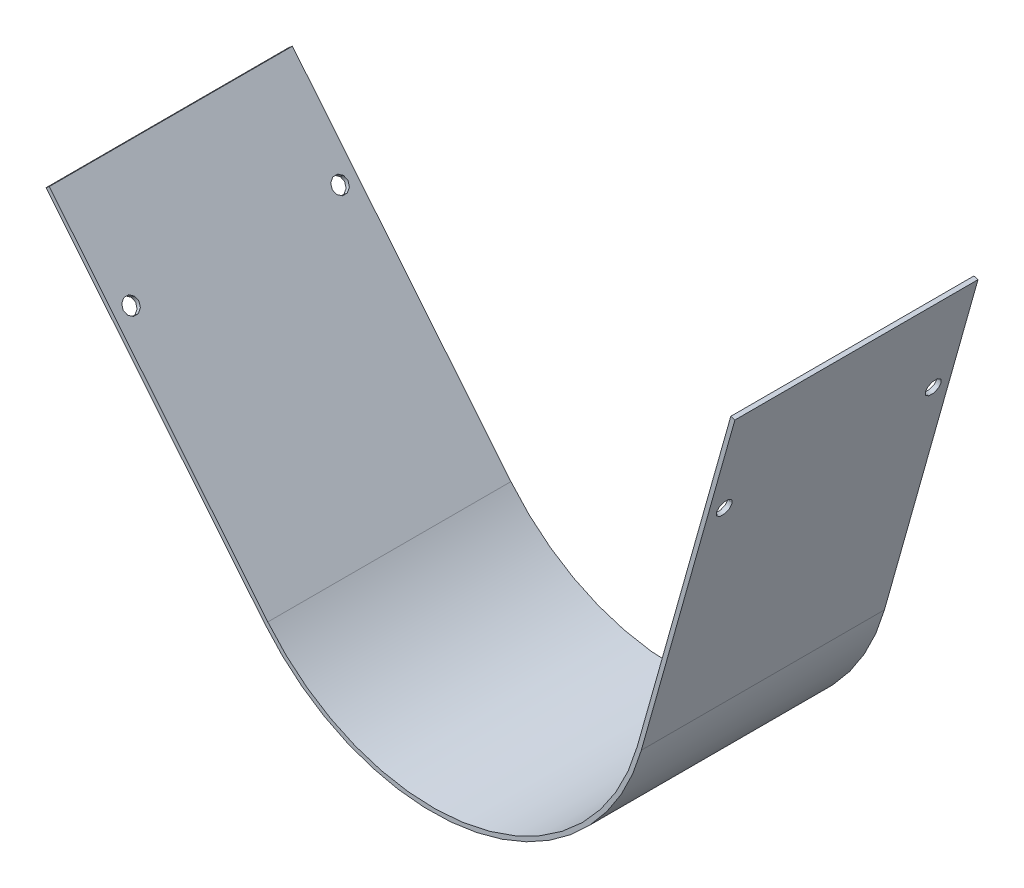
# Autodesk Inventor part: Part2
Saved by Autodesk Inventor 2014 SP1 (Build 180222100, 222)
## iProperties
Created: 2014-01-05
Part Number: Part2
Material: Aluminum 6061
Document SubType Name: Modeling
Designer: Rauhul Varma
Density: 2.71 g/cm^3
Appearance: Anodized - Black
Mass: 21.1129 g
Surface Area: 200.768 cm^2
Volume: 7.79075 cm^3
Author: Rauhul Varma
Autodesk Inventor part; units mm, degrees
ref_plane "YZ Plane" through (0, 0, 0) normal (1, 0, 0) x (0, 1, 0)
ref_plane "XZ Plane" through (0, 0, 0) normal (0, 1, 0) x (-1, 0, 0)
ref_plane "XY Plane" through (0, 0, 0) normal (0, 0, 1) x (1, 0, 0)
sketch "Main Outline" plane through (0, 0, 0) normal (0, 0, 1) x (1, 0, 0)
  line L0 (0, 0) -> (304.8, 0) construction
  line L1 (304.8, 0) -> (304.8, 50.8) construction
  line L2 (304.8, 50.8) -> (0, 50.8) construction
  line L3 (0, 50.8) -> (0, 0) construction
  line L4 (0, 50.8) -> (0, 53.34) construction
  line L5 (0, 53.34) -> (304.8, 53.34) construction
  line L6 (304.8, 53.34) -> (304.8, 50.8) construction
  circle A0 centre (152.4, 23.8125) radius 17.4625 construction
  line L7 (152.4, 23.8125) -> (152.4, 0) construction
  circle A1 centre (152.4, 23.8125) radius 27.94 construction
  circle A2 centre (152.4, 23.8125) radius 21.59 construction
  line L8 (152.4, 23.8125) -> (144.7964, 60.3681) construction
  circle A3 centre (144.7964, 60.3681) radius 15.24 construction
  circle A4 centre (144.7964, 60.3681) radius 8.89 construction
  circle A5 centre (144.7964, 60.3681) radius 14.2875 construction
  arc A6 (164.6591, 71.8014) -> (129.0153, 43.7486) centre (144.7964, 60.3681) ccw construction
  circle A7 centre (98.8106, 85.598) radius 32.258 construction
  circle A8 centre (126.6733, 147.4971) radius 32.258 construction
  circle A9 centre (176.9075, 101.8424) radius 32.258 construction
  circle A10 centre (144.7964, 60.3681) radius 11.1125 construction
  circle A11 centre (152.4, 23.8125) radius 49.53 construction
  line L9 (144.7964, 60.3681) -> (126.6733, 147.4971) construction
  line L10 (144.7964, 60.3681) -> (98.8106, 85.598) construction
  line L11 (98.8106, 85.598) -> (176.9075, 101.8424) construction
  line L12 (176.9075, 101.8424) -> (144.7964, 60.3681) construction
  circle A12 centre (98.8106, 85.598) radius 9.5493 construction
  arc A13 (174.9629, 111.1915) -> (185.6989, 98.1139) centre (176.9075, 101.8424) ccw construction
  circle A14 centre (126.6733, 147.4971) radius 9.5493 construction
  line L13 (96.8659, 94.9472) -> (174.9629, 111.1915) construction
  line L14 (185.6989, 98.1139) -> (165.8956, 51.4198) construction
  line L15 (92.2351, 78.6732) -> (129.0153, 43.7486) construction
  line L16 (174.9629, 111.1915) -> (176.9075, 101.8424) construction
  line L17 (176.9075, 101.8424) -> (185.6989, 98.1139) construction
  arc A15 (185.6989, 98.1139) -> (174.9629, 111.1915) centre (176.9075, 101.8424) ccw construction
  arc A16 (165.8956, 51.4198) -> (164.6591, 71.8014) centre (144.7964, 60.3681) ccw construction
  arc A17 (129.0153, 43.7486) -> (165.8956, 51.4198) centre (144.7964, 60.3681) ccw construction
  circle A18 centre (126.6086, 147.808) radius 32.258 construction
  circle A19 centre (126.544, 148.1188) radius 32.258 construction
  circle A20 centre (126.4793, 148.4297) radius 32.258 construction
  line L18 (126.6733, 147.4971) -> (126.4793, 148.4297) construction
  circle A21 centre (126.738, 147.1863) radius 32.258 construction
  circle A22 centre (117.4622, 43.2997) radius 9.525 construction
  circle A23 centre (176.6694, 55.615) radius 9.525 construction
  line L19 (152.4, 23.8125) -> (117.4622, 43.2997) construction
  line L20 (152.4, 23.8125) -> (176.6694, 55.615) construction
  line L21 (117.4622, 43.2997) -> (98.8106, 85.598) construction
  line L22 (176.6694, 55.615) -> (176.9075, 101.8424) construction
  circle A24 centre (135.1821, 106.5897) radius 7.9375 construction
  line L23 (135.6243, 150.8242) -> (166.2787, 68.353) construction
  circle A25 centre (152.4, 23.8125) radius 29.845 construction
  line L24 (117.1381, 146.979) -> (121.9118, 59.1246) construction
  circle A26 centre (99.0889, 85.4453) radius 32.258 construction
  circle A27 centre (97.9755, 86.0562) radius 32.258 construction
  line L25 (97.9755, 86.0562) -> (98.8106, 85.598) construction
  circle A28 centre (98.2538, 85.9034) radius 32.258 construction
  circle A29 centre (98.5322, 85.7507) radius 32.258 construction
  circle A30 centre (152.4, 23.8125) radius 29.845 construction
  circle A31 centre (122.555, 23.8125) radius 6.35 construction
  circle A32 centre (179.7696, 35.7133) radius 6.35 construction
  line L26 (122.555, 23.8125) -> (152.4, 23.8125) construction
  line L27 (152.4, 23.8125) -> (182.245, 23.8125) construction
  circle A33 centre (182.245, 23.8125) radius 6.35 construction
  circle A34 centre (125.0304, 11.9117) radius 6.35 construction
  circle A35 centre (150.4199, 33.3321) radius 39.5684 construction
  line L28 (72.9795, 65.6655) -> (119.7593, 8.3204) construction
  circle A36 centre (177.4906, 102.5955) radius 32.258 construction
  line L29 (176.9075, 101.8424) -> (177.4906, 102.5955) construction
  circle A37 centre (177.2963, 102.3445) radius 32.258 construction
  circle A38 centre (177.1019, 102.0934) radius 32.258 construction
  circle A39 centre (176.7131, 101.5913) radius 32.258 construction
  line L30 (188.5109, 22.6209) -> (208.5442, 93.8632) construction
  circle A40 centre (135.1821, 106.5897) radius 9.5727 construction
  arc A41 (86.8202, 116.3239) -> (96.3065, 136.4856) centre (81.3304, 131.2195) ccw construction
  arc A42 (158.9123, 149.5077) -> (175.6513, 134.801) centre (174.7462, 150.6502) ccw construction
  line L31 (126.4793, 148.4297) -> (126.9966, 145.9429) construction
  line L32 (116.5322, 146.3607) -> (117.0495, 143.8739) construction
  line L33 (136.9437, 148.0119) -> (136.4264, 150.4987) construction
  arc A43 (136.4264, 150.4987) -> (116.5322, 146.3607) centre (126.4793, 148.4297) ccw construction
  arc A44 (117.0495, 143.8739) -> (136.9437, 148.0119) centre (126.9966, 145.9429) ccw construction
  line L34 (177.4906, 102.5955) -> (175.9357, 100.5871) construction
  line L35 (169.4571, 108.8154) -> (167.9021, 106.807) construction
  line L36 (183.9692, 94.3672) -> (185.5242, 96.3756) construction
  arc A45 (185.5242, 96.3756) -> (169.4571, 108.8154) centre (177.4906, 102.5955) ccw construction
  arc A46 (167.9021, 106.807) -> (183.9692, 94.3672) centre (175.9357, 100.5871) ccw construction
  line L37 (97.9755, 86.0562) -> (100.2023, 84.8344) construction
  line L38 (93.0884, 77.1487) -> (95.3153, 75.927) construction
  line L39 (105.0894, 93.7418) -> (102.8625, 94.9636) construction
  arc A47 (102.8625, 94.9636) -> (93.0884, 77.1487) centre (97.9755, 86.0562) ccw construction
  arc A48 (95.3153, 75.927) -> (105.0894, 93.7418) centre (100.2023, 84.8344) ccw construction
  circle A49 centre (117.4622, 43.2997) radius 3.9687 construction
  circle A50 centre (176.6694, 55.615) radius 3.9687 construction
  line L40 (152.4, 23.8125) -> (158.4777, -5.4071) construction
  arc A51 (80.1751, 59.3139) -> (79.0947, 58.1692) centre (79.7097, 58.6709) ccw construction
  arc A52 (205.9254, 84.5503) -> (204.4781, 85.1692) centre (205.1613, 84.7652) ccw construction
  circle A53 centre (152.4, 23.8125) radius 14.224 construction
  circle A54 centre (135.1821, 106.5897) radius 3.9687 construction
  circle A55 centre (156.538, 3.9183) radius 6.35 construction
  circle A56 centre (156.538, 3.9183) radius 2.0828 construction
  circle A57 centre (152.4, 23.8125) radius 20.32 construction
  line L41 (133.1021, 30.1759) -> (152.4, 23.8125) construction
  line L42 (152.4, 23.8125) -> (167.5599, 37.3432) construction
  circle A58 centre (167.5599, 37.3432) radius 2.0828 construction
  circle A59 centre (167.5599, 37.3432) radius 3.9687 construction
  circle A60 centre (133.1021, 30.1759) radius 2.0828 construction
  circle A61 centre (133.1021, 30.1759) radius 3.9688 construction
  point P0 (126.738, 147.1863)
  point P1 (176.7131, 101.5913)
  dimension "d18" = 99.06
  dimension "d58" = 64.516
  dimension "d86" = 64.516
  dimension "d0" = 304.8
  dimension "d1" = 50.8
  dimension "d2" = 2.54
  dimension "d3" = 34.925
  dimension "d4" = 23.8125
  dimension "d5" = 152.4
  dimension "d6" = 55.88
  dimension "d7" = 43.18
  dimension "d8" = 37.338
  dimension "d10" = 30.48
  dimension "d11" = 17.78
  dimension "d12" = 28.575
  dimension "d13" = 45.8366
  dimension "d14" = 64.516
  dimension "d15" = 64.516
  dimension "d16" = 64.516
  dimension "d17" = 22.225
  dimension "d19" = 52.4523
  dimension "d20" = 88.9939
  dimension "d21" = 19.0986
  dimension "d22" = 19.0986
  dimension "d23" = 19.0986
  dimension "d30" = 124.732
  dimension "d40" = 64.516
  dimension "d41" = 64.516
  dimension "d42" = 64.516
  dimension "d43" = 0.9525
  dimension "d44" = 0.3175
  dimension "d45" = 0.635
  dimension "d46" = 64.516
  dimension "d47" = 0.3175
  dimension "d48" = 19.05
  dimension "d49" = 19.05
  dimension "d50" = 40.005
  dimension "d51" = 40.005
  dimension "d52" = 46.228
  dimension "d54" = 46.228
  dimension "d55" = 15.875
  dimension "d56" = 41.4655
  dimension "d57" = 59.69
  dimension "d59" = 64.516
  dimension "d60" = 64.516
  dimension "d61" = 64.516
  dimension "d62" = 0.3175
  dimension "d63" = 0.3175
  dimension "d64" = 0.635
  dimension "d65" = 0.9525
  dimension "d73" = 12.7
  dimension "d74" = 12.7
  dimension "d76" = 59.69
  dimension "d78" = 12.7
  dimension "d79" = 12.7
  dimension "d80" = 64.516
  dimension "d81" = 0.9525
  dimension "d82" = 64.516
  dimension "d83" = 64.516
  dimension "d84" = 0.3175
  dimension "d85" = 0.635
  dimension "d88" = 0.3175
  dimension "d89" = 31.75
  dimension "d90" = 31.75
  dimension "d94" = 1.5875
  dimension "d95" = 20.32
  dimension "d96" = 1.5875
  constraints: 92 end point, 59 centre point, 54 point on circle, 38 tangent, 26 coincident, 16 point on line, 9 collinear, 6 parallel, 4 midpoint, 4 perpendicular, 3 symmetric about line, 2 horizontal, 13 other
  measures "d0" distance of L2.end L1.end
  measures "d1" distance of L1.end L0.end
  measures "d2" distance of L2.end L4.end
  measures "d3" diameter of A0
  measures "d4" distance of L7.start L7.end
  measures "d5" distance between parallel lines of L3 L7
  measures "d6" diameter of A1
  measures "d7" diameter of A2
  measures "d8" distance of L8.start L8.end
  measures "d10" diameter of A3
  measures "d11" diameter of A4
  measures "d12" diameter of A5
  measures "d13" diameter of A6
  measures "d14" diameter of A7
  measures "d15" diameter of A8
  measures "d16" diameter of A9
  measures "d17" diameter of A10
  measures "d19" distance of L9.start L10.end
  measures "d20" distance of L9.start L9.end
  measures "d21" diameter of A12
  measures "d22" diameter of A13
  measures "d23" diameter of A14
  measures "d30" angle of L17 L16
  measures "d40" diameter of A18
  measures "d41" diameter of A19
  measures "d42" diameter of A20
  measures "d43" distance of L18.end L9.end
  measures "d44" distance of A18.centre L9.end
  measures "d45" distance of A19.centre L9.end
  measures "d46" diameter of A21
  measures "d47" distance of L9.end A21.centre
  measures "d48" diameter of A22
  measures "d49" diameter of A23
  measures "d50" distance of L19.start L19.end
  measures "d51" distance of L19.start L20.end
  measures "d52" distance of L19.end L21.end
  measures "d54" distance of L20.end L16.end
  measures "d55" diameter of A24
  measures "d56" distance of A21.centre A24.centre
  measures "d57" diameter of A25
  measures "d59" diameter of A27
  measures "d60" diameter of A28
  measures "d61" diameter of A29
  measures "d62" distance of point (99.089, 85.445) L10.end
  measures "d63" distance of L10.end A29.centre
  measures "d64" distance of L10.end A28.centre
  measures "d65" distance of L25.start L10.end
  measures "d73" diameter of A31
  measures "d74" diameter of A32
  measures "d76" diameter of A30
  measures "d78" diameter of A33
  measures "d79" diameter of A34
  measures "d80" diameter of A36
  measures "d81" distance of L29.start L29.end
  measures "d82" diameter of A37
  measures "d83" diameter of A38
  measures "d84" distance of L16.end A38.centre
  measures "d85" distance of L11.end A37.centre
  measures "d88" distance of L11.end point (176.713, 101.591)
  measures "d89" diameter of A41
  measures "d90" diameter of A42
  measures "d94" distance of L9.end L31.end
  measures "d95" diameter of A44
  measures "d96" distance of L11.end L34.end
sketch "Upper CIM C-C Check" plane through (0, 0, 0) normal (0, 0, 1) x (1, 0, 0)
  arc A0 (3.4429, -22.6582) -> (3.4429, 22.6582) centre (0, 0) ccw construction
  arc A1 (90.4285, 9.4409) -> (90.4285, -9.4409) centre (88.9939, 0) ccw construction
  line L0 (88.9939, 0) -> (0, 0) construction
  line L1 (90.4285, 9.4409) -> (3.4429, 22.6582)
  line L2 (3.4429, -22.6582) -> (90.4285, -9.4409)
  arc A2 (90.4285, -9.4409) -> (90.4285, 9.4409) centre (88.9939, 0) ccw
  arc A3 (3.4429, 22.6582) -> (3.4429, -22.6582) centre (0, 0) ccw
  dimension "d24" = 45.8366
  dimension "d25" = 19.0986
  dimension "d26" = 78.9119
  dimension "d27" = 87.984
  dimension "d28" = 27.12
  dimension "d29" = 88.9939
  constraints: 8 point on circle, 6 end point, 4 centre point, 4 tangent, 1 coincident, 1 horizontal
  measures "d24" diameter of A0
  measures "d25" diameter of A1
  measures "d27" distance of L1.start L1.end
  measures "d29" distance of L0.start L0.end
sketch "Sketch3" plane through (0, 0, 0) normal (0, 0, 1) x (1, 0, 0)
  arc A0 (80.1751, 59.3139) -> (79.0947, 58.1692) centre (79.7097, 58.6709) ccw construction
  line L0 (72.9795, 65.6655) -> (119.7593, 8.3204) construction
  circle A1 centre (150.4199, 33.3321) radius 39.5684 construction
  line L1 (188.5109, 22.6209) -> (208.5442, 93.8632) construction
  arc A2 (205.9254, 84.5503) -> (204.4781, 85.1692) centre (205.1613, 84.7652) ccw construction
  line L2 (79.0947, 58.1692) -> (119.7593, 8.3204)
  line L3 (188.5109, 22.6209) -> (205.9254, 84.5503)
  arc A3 (119.7593, 8.3204) -> (188.5109, 22.6209) centre (150.4199, 33.3321) ccw
  line L4 (78.4796, 57.6675) -> (119.1442, 7.8187)
  arc A4 (119.1442, 7.8187) -> (189.275, 22.4061) centre (150.4199, 33.3321) ccw
  line L5 (189.275, 22.4061) -> (206.6896, 84.3354)
  line L6 (79.0947, 58.1692) -> (78.4796, 57.6675)
  line L7 (206.6896, 84.3354) -> (205.9254, 84.5503)
  point P0 (0, 0)
  dimension "d115" = 0.7937
  constraints: 12 end point, 4 point on circle, 4 tangent, 2 centre point, 2 collinear, 2 perpendicular, 1 coincident, 2 other
  measures "d115" distance between parallel lines of L0 L4
extrude "Extrusion1" add sketch "Sketch3" along normal blind 45.2437
ref_plane "Work Plane1" through (144.7964, 60.3681, 0) normal (0.9790451, 0.2036437, 0) x (-0.2036437, 0.9790451, 0)
sketch "Sketch4" plane through (188.5109, 22.6209, 0) normal (-0.9626636, 0.2707007, 0) x (0, 0, 1)
  line L0 (0, 0) -> (0, 64.3313) projected
  line L1 (0, 0) -> (45.2437, 0) projected
  line L2 (45.2437, 64.3313) -> (45.2437, 0) projected
  line L3 (0, 64.3313) -> (45.2437, 64.3313) projected
  line L4 (3.175, 64.3313) -> (3.175, 0)
  line L5 (42.0688, 64.3313) -> (42.0688, 0)
  point P0 (0, -72.8064)
  point P1 (3.175, 45.2813)
  point P2 (42.0688, 45.2813)
  dimension "d119" = 3.175
  dimension "d120" = 3.175
  dimension "d121" = 19.05
  dimension "d122" = 19.05
  constraints: 6 point on line, 4 end point, 2 perpendicular
  measures "d119" distance between parallel lines of L0 L4
  measures "d120" distance between parallel lines of L2 L5
  measures "d121" distance from line of L3 point (3.175, 45.281)
  measures "d122" distance from line of L3 point (42.069, 45.281)
hole "Hole1" at (200.7686, 66.2116, 3.175) at (200.7686, 66.2116, 42.0688) direction (0.9626636, -0.2707007, 0) diameter 2.9464 end through all clearance for "Flat Head Machine Screw (82)" size "#4" standard "Ansi Unified Screw Threads"
mirror "Mirror1" about plane through (144.7964, 60.3681, 0) normal (0.9790451, 0.2036437, 0) of "Hole1"
sketch "Sketch6" plane through (0, 0, 45.2437) normal (0, 0, 1) x (1, 0, 0)
  line L0 (119.7593, 8.3204) -> (79.0947, 58.1692) projected
  line L1 (79.0947, 58.1692) -> (78.4796, 57.6675) projected
  line L2 (78.4796, 57.6675) -> (119.1442, 7.8187) projected
  arc A0 (119.1442, 7.8187) -> (189.275, 22.4061) centre (150.4199, 33.3321) ccw projected
  line L3 (189.275, 22.4061) -> (206.6896, 84.3354) projected
  line L4 (206.6896, 84.3354) -> (205.9254, 84.5503) projected
  line L5 (205.9254, 84.5503) -> (188.5109, 22.6209) projected
  arc A1 (119.7593, 8.3204) -> (188.5109, 22.6209) centre (150.4199, 33.3321) ccw projected
  line L6 (46.0816, -65.5817) -> (259.8786, -42.4203)
  point P0 (0, 0)
  dimension "d135" = 86.3855
  dimension "d136" = 64.3312
  dimension "d137" = 215.048
  constraints: 2 end point
  measures "d136" distance of L0.start L0.end
  measures "d137" distance of L6.start L6.end
equation "\"d3\" = r10"
equation "\"d6\" = g44"
equation "\"d7\" = g34"
equation "\"d10\" = g24"
equation "\"d11\" = g14"
equation "\"d12\" = r8"
equation "\"d13\" = p48"
equation "\"d14\" = cim"
equation "\"d15\" = cim"
equation "\"d16\" = cim"
equation "\"d17\" = r6"
equation "\"d21\" = p20"
equation "\"d22\" = p20"
equation "\"d23\" = p20"
equation "\"d24\" = p48"
equation "\"d25\" = p20"
equation "\"d29\" = d20"
equation "\"g14\" = 17.78"
equation "\"g24\" = 30.48"
equation "\"g34\" = 43.18"
equation "\"g44\" = 55.88"
equation "\"p20\" = 19.09859"
equation "\"p48\" = 45.83662"
equation "\"r10\" = 34.925"
equation "\"r9\" = 31.75"
equation "\"r8\" = 28.575"
equation "\"r7\" = 25.4"
equation "\"r6\" = 22.225"
equation "\"r5\" = 19.05"
equation "\"r4\" = 15.875"
equation "\"r3\" = 12.7"
equation "\"cim\" = 64.516"
equation "\"act\" = 28.448"
equation "\"actL\" = 23.749"
equation "\"UpperCimCCCheck\" = 2 * d27 + d26 + d28"
equation "\"LowerBeltPathCCCheck\" = 267"
equation "\"SheildArc\" = 215.04798"
body "Solid1"
